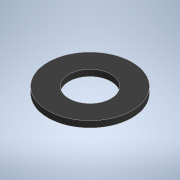
# Autodesk Inventor part: Pump-Motor-CW-Rotation:Gasket 102
Saved by Autodesk Inventor 2022.2 (Build 262287010, 287A)
## iProperties
Created: 2025-06-16
Material: Rubber, Silicone
Document SubType Name: Modeling
Density: 1.25 g/cm^3
Appearance: Rubber - Black
Designer: cw
Author: cw
Autodesk Inventor part; units mm, degrees
ref_plane "YZ Plane" through (0, 0, 0) normal (1, 0, 0) x (0, 1, 0)
ref_plane "XZ Plane" through (0, 0, 0) normal (0, 1, 0) x (-1, 0, 0)
ref_plane "XY Plane" through (0, 0, 0) normal (0, 0, 1) x (1, 0, 0)
sketch "Sketch1" plane through (0, 0, 0) normal (0, 0, 1) x (1, 0, 0)
  circle A0 centre (0, 0) radius 10
  circle A1 centre (0, 0) radius 5
  dimension "d0" = 20
  dimension "d1" = 10
  constraints: 2 centre point, 2 coincident
  measures "d0" diameter of A0
  measures "d1" diameter of A1
extrude "Extrusion1" add sketch "Sketch1" along normal mid plane 1.5
body "Solid1"
